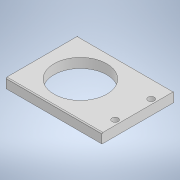
# Autodesk Inventor part: blok_łożyska
Saved by Autodesk Inventor 2020 (Build 240168000, 168)
## iProperties
Created: 2020-08-17
Part Number: blok_łożyska
Material: Generic
Document SubType Name: Modeling
Designer: Hesekiel
Density: 1 g/cm^3
Appearance: Default
Author: Hesekiel
Autodesk Inventor part; units mm, degrees
ref_plane "YZ Plane" through (0, 0, 0) normal (1, 0, 0) x (0, 1, 0)
ref_plane "XZ Plane" through (0, 0, 0) normal (0, 1, 0) x (-1, 0, 0)
ref_plane "XY Plane" through (0, 0, 0) normal (0, 0, 1) x (1, 0, 0)
sketch "Sketch1" plane through (0, 0, 0) normal (0, 1, 0) x (-1, 0, 0)
  line L0 (-50, 37.5) -> (50, 37.5)
  line L1 (50, 37.5) -> (50, -37.5)
  line L2 (50, -37.5) -> (-50, -37.5)
  line L3 (-50, -37.5) -> (-50, 37.5)
  line L4 (-50, 37.5) -> (50, -37.5) construction
  line L5 (50, 37.5) -> (-50, -37.5) construction
  line L6 (50, 0) -> (10, 0)
  circle A0 centre (10, 0) radius 27.5
  point P0 (0, 0)
  dimension "d0" = 100
  dimension "d1" = 75
  dimension "d2" = 40
  dimension "d3" = 55
  constraints: 14 end point, 3 midpoint, 2 horizontal, 2 parallel, 1 centre point, 1 coincident, 1 perpendicular
  measures "d0" distance of L1.end L2.end
  measures "d1" distance of L0.end L1.end
  measures "d2" distance of L6.start L6.end
  measures "d3" diameter of A0
extrude "Extrusion1" add sketch "Sketch1" along normal blind 10
sketch "Sketch2" plane through (0, 10, 0) normal (0, 1, 0) x (1, 0, 0)
  line L0 (50, 37.5) -> (-50, 37.5) projected
  line L1 (-50, -37.5) -> (50, -37.5) projected
  line L2 (50, 37.5) -> (40, 37.5)
  line L3 (40, 37.5) -> (40, -37.5)
  line L4 (40, -37.5) -> (50, -37.5)
  line L5 (50, -37.5) -> (50, 37.5)
  line L6 (45, 37.5) -> (45, 0)
  line L7 (45, 0) -> (45, -37.5)
  circle A0 centre (45, 18.75) radius 3.3
  circle A1 centre (45, -18.75) radius 3.3
  point P0 (0, 0)
  dimension "d6" = 10
  dimension "d7" = 6.6
  dimension "d8" = 6.6
  constraints: 12 end point, 4 midpoint, 2 centre point, 2 parallel, 1 horizontal, 1 perpendicular, 1 point on line, 1 vertical
  measures "d6" distance of L4.end L3.end
  measures "d7" diameter of A0
  measures "d8" diameter of A1
extrude "Extrusion2" cut sketch "Sketch2" against normal up to surface (10 mm away) contours A0 L6 | L6 A0 | A1 L7 | L7 A1
fillet "Fillet1" radius 1 2 edges at (0, 10, 37.5) (0, 10, -37.5)
body "Solid1"
